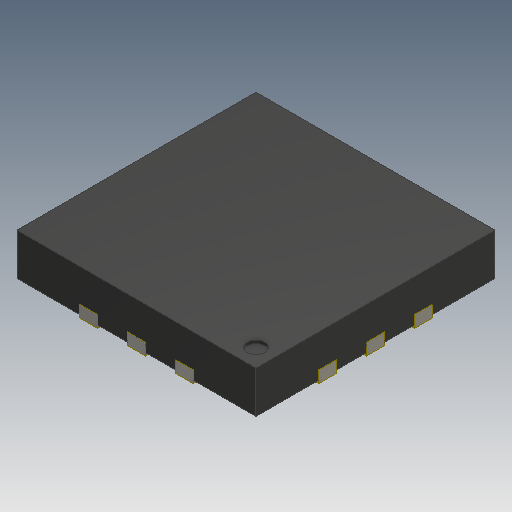
# Autodesk Inventor part: qfn-12
Saved by Autodesk Inventor 2017 (Build 210142000, 142)
## iProperties
Created: 2015-10-12
Part Number: qfn-12
Material: ABS Plastic
Document SubType Name: Modeling
Designer: Sawaiz
Density: 1.06 g/cm^3
Appearance: Smooth - Black
width: 4.000 mm
length: 4.000 mm
height: 0.750 mm
leadFrame: 0.200 mm
seatingHeight: 0.050 mm
padSpacing: 0.800 mm
padDepth: 0.500 mm
padWidth: 0.300 mm
numLeads: 12.000 ul
Author: Sawaiz
Autodesk Inventor part; units mm, degrees
ref_plane "YZ Plane" through (0, 0, 0) normal (1, 0, 0) x (0, 1, 0)
ref_plane "XZ Plane" through (0, 0, 0) normal (0, 1, 0) x (-1, 0, 0)
ref_plane "XY Plane" through (0, 0, 0) normal (0, 0, 1) x (1, 0, 0)
sketch "Sketch1" plane through (0, 0, 0) normal (0, 0, 1) x (1, 0, 0)
  line L0 (2, -2) -> (-2, -2)
  line L1 (-2, -2) -> (-2, 2)
  line L2 (-2, 2) -> (2, 2)
  line L3 (2, 2) -> (2, -2)
  line L4 (2, -2) -> (-2, 2) construction
  line L5 (-2, -2) -> (2, 2) construction
  point P0 (0, 0)
  dimension "d0" = 4
  dimension "d1" = 4
  constraints: 12 end point, 2 midpoint, 2 parallel, 1 horizontal, 1 perpendicular
  measures "d0" distance of L1.end L2.end
  measures "d1" distance of L0.end L1.end
extrude "Extrusion1" add sketch "Sketch1" along normal blind 0.7
sketch "Sketch2" plane through (0, 0, 0) normal (0, 0, -1) x (-1, 0, 0)
  line L0 (-2, -2) -> (2, -2) projected
  line L1 (2, -2) -> (2, 2) projected
  line L2 (2, 2) -> (-2, 2) projected
  line L3 (-2, 2) -> (-2, -2) projected
  line L4 (0, 0) -> (-2, 0)
  circle A0 centre (-1.65, 0) radius 0.15
  line L5 (-1.65, 0.15) -> (-2, 0.15)
  line L6 (-1.65, -0.15) -> (-2, -0.15)
  line L7 (-2, -2) -> (-2, 2) projected
  dimension "d4" = 0.3
  dimension "d5" = 0.35
  constraints: 6 end point, 3 point on line, 2 point on circle, 2 tangent, 1 centre point, 1 midpoint, 1 parallel, 1 perpendicular
  measures "d4" diameter of A0
  measures "d5" distance from line of L3 A0.centre
extrude "Extrusion2" cut sketch "Sketch2" against normal blind 0.15 contours L3 L4 A0 L6 | L3 L5 A0 L4 | A0 L4 | A0 L4
sketch "Sketch3" plane through (0, 0, 0) normal (0, 0, -1) x (-1, 0, 0)
  line L0 (-1.2, -1.2) -> (1.2, -1.2)
  line L1 (1.2, -1.2) -> (1.2, 1.2)
  line L2 (1.2, 1.2) -> (-0.825, 1.2)
  line L3 (-1.2, 0.825) -> (-1.2, -1.2)
  line L4 (-1.2, -1.2) -> (1.2, 1.2) construction
  line L5 (1.2, -1.2) -> (-1.2, 1.2) construction
  line L6 (-0.825, 1.2) -> (-1.2, 0.825)
  point P0 (0, 0)
  dimension "d14" = 2.4
  dimension "d15" = 2.4
  dimension "d16" = 0.375
  dimension "d17" = 0.375
  constraints: 14 end point, 2 midpoint, 2 parallel, 2 point on line, 1 horizontal, 1 perpendicular
  measures "d14" distance of L5.end L1.end
  measures "d15" distance of L1.end L0.end
  measures "d16" distance of L2.end L5.end
  measures "d17" distance of L3.start L5.end
extrude "Extrusion3" add sketch "Sketch3" along normal blind 0.05
sketch "Sketch5" plane through (0, 0, 0.7) normal (0, 0, 1) x (1, 0, 0)
  circle A0 centre (1.7, 1.7) radius 0.15
  line L0 (2, -2) -> (2, 2) projected
  line L1 (2, 2) -> (-2, 2) projected
  point P0 (0, 0)
  dimension "d29" = 0.3
  dimension "d30" = 0.3
  dimension "d31" = 0.3
  constraints: 1 centre point
  measures "d29" diameter of A0
  measures "d30" distance from line of L0 A0.centre
  measures "d31" distance from line of L1 A0.centre
extrude "Extrusion5" cut sketch "Sketch5" against normal blind 0.05
pattern_linear "Rectangular Pattern3" count 3 spacing 0.8 along (0, -1, 0) of "Extrusion2" first direction both ways yes
mirror "Mirror1" about plane through (0, 0, 0) normal (1, 0, 0) of "Extrusion2", "Rectangular Pattern3"
sketch "Sketch6" plane through (0, 0, 0) normal (0, 0, -1) x (-1, 0, 0)
  line L0 (2, 2) -> (-2, 2) projected
  circle A0 centre (0, 1.65) radius 0.15
  line L1 (-0.15, 1.65) -> (-0.15, 2)
  line L2 (0.15, 1.65) -> (0.15, 2)
  line L3 (-2, 2) -> (2, 2) projected
  point P0 (0, 0)
  point P1 (0, 2)
  dimension "d37" = 0.3
  dimension "d38" = 0.35
  dimension "d64" = 0
  constraints: 4 end point, 2 point on circle, 2 point on line, 2 tangent, 1 centre point, 1 midpoint, 1 perpendicular, 1 vertical
  measures "d37" diameter of A0
  measures "d38" distance from line of L0 A0.centre
  measures "d64" horizontal distance of A0.centre point (0, 2)
extrude "Extrusion6" cut sketch "Sketch6" against normal blind 0.15
pattern_linear "Rectangular Pattern4" count 3 spacing 0.8 along (1, 0, 0) of "Extrusion6" first direction both ways yes
mirror "Mirror2" about plane through (0, 0, 0) normal (0, 1, 0) of "Extrusion6", "Rectangular Pattern4"
sketch "Sketch7" plane through (0, 0, 0.15) normal (0, 0, -1) x (-1, 0, 0)
  line L0 (-1.65, -0.15) -> (-2, -0.15) projected
  arc A0 (-1.65, -0.15) -> (-1.65, 0.15) centre (-1.65, 0) ccw projected
  line L1 (-2, 0.15) -> (-1.65, 0.15) projected
  line L2 (-2, -0.15) -> (-2, 0.15) projected
  point P0 (0, 0)
extrude "Extrusion7" add sketch "Sketch7" along normal blind 0.2 separate body
pattern_linear "Rectangular Pattern5" count 3 spacing 0.8 along (0, -1, 0) of "Extrusion7" first direction both ways yes bodies 2
sketch "Sketch8" plane through (-1.65, -0.15, 0.15) normal (0, 0, -1) x (-1, 0, 0)
  line L0 (0, 0) -> (0.35, 0) projected
  line L1 (0.35, 0.3) -> (0.35, 0) projected
  line L2 (0.35, 0.3) -> (0, 0.3) projected
  arc A0 (0, 0.3) -> (0, 0) centre (0, 0.15) ccw projected
  point P0 (-1.65, 0.15)
extrude "Extrusion8" add sketch "Sketch8" along normal blind 0.2 separate body
pattern_linear "Rectangular Pattern6" count 3 spacing 0.8 along (0, 1, 0) of "Extrusion8" first direction both ways yes bodies 3
sketch "Sketch9" plane through (0, 0, 0.15) normal (0, 0, -1) x (-1, 0, 0)
  arc A0 (-0.15, 1.65) -> (0.15, 1.65) centre (0, 1.65) ccw projected
  line L0 (0.15, 2) -> (0.15, 1.65) projected
  line L1 (-0.15, 2) -> (0.15, 2) projected
  line L2 (-0.15, 1.65) -> (-0.15, 2) projected
  point P0 (0, 0)
extrude "Extrusion9" add sketch "Sketch9" along normal blind 0.2 separate body
pattern_linear "Rectangular Pattern7" count 3 spacing 0.8 along (1, 0, 0) of "Extrusion9" first direction both ways yes bodies 4
sketch "Sketch10" plane through (0, -1.65, 0.15) normal (0, 0, -1) x (-1, 0, 0)
  arc A0 (0.15, 0) -> (-0.15, 0) centre (0, 0) ccw projected
  line L0 (-0.15, 0) -> (-0.15, -0.35) projected
  line L1 (0.15, -0.35) -> (-0.15, -0.35) projected
  line L2 (0.15, -0.35) -> (0.15, 0) projected
  point P0 (0, 1.65)
extrude "Extrusion10" add sketch "Sketch10" along normal blind 0.2 separate body
pattern_linear "Rectangular Pattern8" count 3 spacing 0.8 along (-1, 0, 0) of "Extrusion10" first direction both ways yes bodies 5
equation "\"d0\" = width"
equation "\"d1\" = length"
equation "\"d2\" = height - seatingHeight"
equation "\"d4\" = padWidth"
equation "\"d5\" = padDepth - 0.5 * padWidth"
equation "\"d6\" = leadFrame - seatingHeight"
equation "\"d14\" = 0.6 * width"
equation "\"d15\" = 0.6 * length"
equation "\"d16\" = 0.5 * height"
equation "\"d17\" = d16"
equation "\"d18\" = seatingHeight"
equation "\"d29\" = 0.4 * height"
equation "\"d30\" = 0.4 * height"
equation "\"d31\" = 0.4 * height"
equation "\"d32\" = seatingHeight"
equation "\"d36\" = padSpacing"
equation "\"d37\" = padWidth"
equation "\"d38\" = padDepth - 0.5 * padWidth"
equation "\"d39\" = leadFrame - seatingHeight"
equation "\"d43\" = padSpacing"
equation "\"d44\" = leadFrame"
equation "\"d48\" = padSpacing"
equation "\"d49\" = leadFrame"
equation "\"d53\" = padSpacing"
equation "\"d54\" = leadFrame"
equation "\"d58\" = padSpacing"
equation "\"d59\" = leadFrame"
equation "\"d63\" = padSpacing"
equation "\"width\" = 4"
equation "\"length\" = 4"
equation "\"height\" = 0.75"
equation "\"leadFrame\" = 0.2"
equation "\"seatingHeight\" = 0.05"
equation "\"padSpacing\" = 0.8"
equation "\"padDepth\" = 0.5"
equation "\"padWidth\" = 0.3"
equation "\"numLeads\" = 12"
body "Solid1"
body "Solid2"
body "Solid3"
body "Solid4"
body "Solid5"
